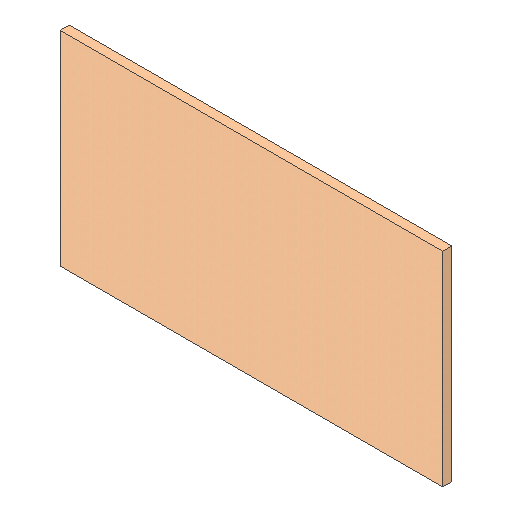
# Autodesk Inventor part: CNCM_WOOD_18mm_Base_plate
Saved by Autodesk Inventor 2026.1 (Build 301233000, 233)
## iProperties
Created: 2018-06-16
Part Number: CNCM_WOOD_18mm_Base_plate
Material: Wood (Birch)
Document SubType Name: Modeling
Designer: Andrzej
Density: 0.55 g/cm^3
Appearance: White Oak
Author: Andrzej
Autodesk Inventor part; units mm, degrees
ref_plane "YZ Plane" through (0, 0, 0) normal (1, 0, 0) x (0, 1, 0)
ref_plane "XZ Plane" through (0, 0, 0) normal (0, 1, 0) x (-1, 0, 0)
ref_plane "XY Plane" through (0, 0, 0) normal (0, 0, 1) x (1, 0, 0)
sketch "Sketch1" plane through (0, 0, 0) normal (0, 0, 1) x (1, 0, 0)
  line L0 (-375, 200) -> (375, 200)
  line L1 (375, 200) -> (375, -200)
  line L2 (375, -200) -> (-375, -200)
  line L3 (-375, -200) -> (-375, 200)
  line L4 (30, 104) -> (238, 104)
  line L5 (238, 104) -> (238, -104)
  line L6 (238, -104) -> (30, -104)
  line L7 (30, -104) -> (30, 104)
  line L8 (40, 94) -> (228, 94)
  line L9 (228, 94) -> (228, -94)
  line L10 (228, -94) -> (40, -94)
  line L11 (40, -94) -> (40, 94)
  point P0 (0, 0)
  point P1 (36, -98)
  point P2 (36, 0)
  point P3 (36, 98)
  point P4 (134, -98)
  point P5 (232, -98)
  point P6 (232, 0)
  point P7 (232, 98)
  point P8 (134, 98)
  dimension "d0" = 750
  dimension "d1" = 400
  dimension "d4" = 208
  dimension "d5" = 208
  dimension "d6" = 96
  dimension "d8" = 375
  dimension "d9" = 200
  dimension "d10" = 137
  dimension "d11" = 10
  dimension "d14" = 6
  dimension "d16" = 6
  dimension "d17" = 6
  dimension "d19" = 104
  dimension "d20" = 6
  dimension "d28" = 104
  constraints: 24 end point, 6 parallel, 5 horizontal alignment, 5 vertical alignment, 3 perpendicular, 2 horizontal, 3 other
  measures "d0" distance of L1.end L2.end
  measures "d1" distance of L0.end L1.end
  measures "d4" distance of L4.start L4.end
  measures "d5" distance of L6.end L4.start
  measures "d6" distance between parallel lines of L2 L6
  measures "d8" distance from line of L3 point (0, 0)
  measures "d9" distance from line of point (0, 0) L2
  measures "d10" distance between parallel lines of L1 L5
  measures "d11" distance between parallel lines of L7 L11
  measures "d14" distance from line of L4 point (36, 98)
  measures "d16" distance from line of L6 point (36, -98)
  measures "d17" distance from line of L7 point (36, -98)
  measures "d19" distance from line of L6 point (36, 0)
  measures "d20" distance from line of L5 point (232, -98)
  measures "d28" distance from line of point (134, -98) L7
extrude "Extrusion1" add sketch "Sketch1" along normal blind 18 contours L0 L1 L2 L3 | L4 L5 L6 L7 | L8 L9 L10 L11
equation "\"d5\" = d4"
equation "\"d6\" = -0.5 * d5 + 0.5 * d1"
equation "\"d8\" = 0.5 * d0"
equation "\"d9\" = 0.5 * d1"
equation "\"d17\" = d16"
equation "\"d20\" = d16"
equation "\"d28\" = d19"
body "Solid1"
